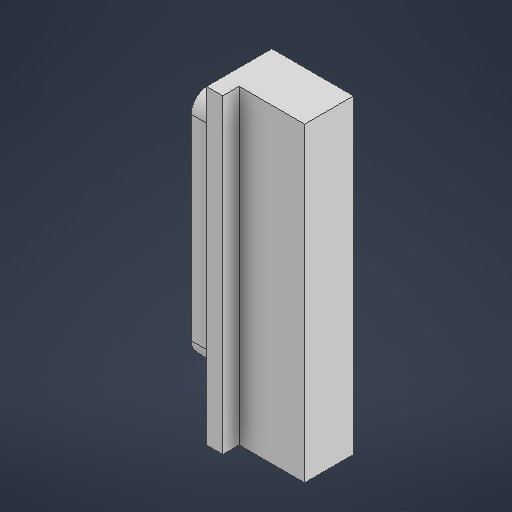
# Autodesk Inventor part: 指纹识别
Saved by Autodesk Inventor 2025 (Build 290162000, 162)
## iProperties
Created: 2025-11-17
Part Number: 指纹识别
Material: 常规
Document SubType Name: Modeling
Designer: XH
Density: 1 g/cm^3
Appearance: 默认
Author: XH
Autodesk Inventor part; units mm, degrees
ref_plane "YZ Plane" through (0, 0, 0) normal (1, 0, 0) x (0, 1, 0)
ref_plane "XZ Plane" through (0, 0, 0) normal (0, 1, 0) x (-1, 0, 0)
ref_plane "XY Plane" through (0, 0, 0) normal (0, 0, 1) x (1, 0, 0)
sketch "草图1" plane through (0, 0, 0) normal (0, 0, 1) x (1, 0, 0)
  line L0 (2.5, -9.5) -> (-2.5, -9.5)
  line L1 (-2.5, -9.5) -> (-2.5, 9.5)
  line L2 (-2.5, 9.5) -> (2.5, 9.5)
  line L3 (2.5, 9.5) -> (2.5, -9.5)
  line L4 (2.5, -9.5) -> (-2.5, 9.5) construction
  line L5 (-2.5, -9.5) -> (2.5, 9.5) construction
  point P0 (0, 0)
  dimension "d0" = 5
  dimension "d1" = 19
  constraints: 12 end point, 2 midpoint, 2 parallel, 1 horizontal, 1 perpendicular
  measures "d0" distance of L1.end L2.end
  measures "d1" distance of L2.end L0.start
extrude "拉伸1" add sketch "草图1" along normal blind 3
sketch "草图2" plane through (0, 0, 3) normal (0, 0, 1) x (1, 0, 0)
  line L0 (2.5, 9.5) -> (-2.5, 9.5) projected
  line L1 (-2.5, -9.5) -> (2.5, -9.5) projected
  line L2 (-2.5, 9.5) -> (-1.5, 9.5)
  line L3 (-1.5, 9.5) -> (-1.5, -9.5)
  line L4 (-1.5, -9.5) -> (-2.5, -9.5)
  line L5 (-2.5, -9.5) -> (-2.5, 9.5)
  point P0 (0, 0)
  dimension "d4" = 1
  constraints: 8 end point, 2 parallel, 1 horizontal, 1 perpendicular, 1 point on line
  measures "d4" distance between parallel lines of L5 L3
extrude "拉伸2" add sketch "草图2" along normal blind 1
sketch "草图3" plane through (-2.5, -9.5, 0) normal (-1, 0, 0) x (0, 0, 1)
  line L0 (0.9436, 15) -> (0.9436, 3) construction
  line L1 (-0.0564, 15) -> (-0.0564, 3)
  line L2 (1.9436, 3) -> (1.9436, 15)
  arc A0 (1.9436, 15) -> (-0.0564, 15) centre (0.9436, 15) ccw
  arc A1 (-0.0564, 3) -> (1.9436, 3) centre (0.9436, 3) ccw
  line L3 (0, 19) -> (4, 19) projected
  point P0 (0, 9.5)
  point P1 (0.9436, 9)
  point P2 (0.9436, 16)
  point P3 (0.9436, 2)
  dimension "d7" = 2
  dimension "d8" = 14
  dimension "d9" = 3
  constraints: 8 end point, 6 point on circle, 4 tangent, 2 centre point, 1 midpoint, 1 parallel, 1 vertical
  measures "d7" distance between parallel lines of L1 L2
  measures "d8" distance of point (0.944, 16) point (0.944, 2)
  measures "d9" distance from line of L3 point (0.944, 16)
extrude "拉伸3" add sketch "草图3" along normal blind 3
